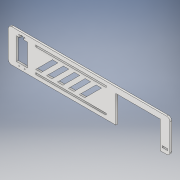
# Autodesk Inventor part: Cuerpo - LateralPrueba
Saved by Autodesk Inventor 2019 (Build 230136000, 136)
## iProperties
Created: 2020-02-14
Part Number: Cuerpo - LateralPrueba
Material: ABS Plastic
Document SubType Name: Modeling
Designer: Mafer1
Density: 1.06 g/cm^3
Appearance: Smooth - White
Mass: 36.6909 g
Surface Area: 287.559 cm^2
Volume: 34.614 cm^3
base_servo: 20.000 mm
altura_servo: 40.000 mm
agujero_servo: 2.000 mm
distancia_agujero_servo: 4.750 mm
largo_base: 200.000 mm
Author: Mafer1
Autodesk Inventor part; units mm, degrees
ref_plane "YZ Plane" through (0, 0, 0) normal (1, 0, 0) x (0, 1, 0)
ref_plane "XZ Plane" through (0, 0, 0) normal (0, 1, 0) x (-1, 0, 0)
ref_plane "XY Plane" through (0, 0, 0) normal (0, 0, 1) x (1, 0, 0)
sketch "Sketch7" plane through (0, 0, 0) normal (0, 0, 1) x (1, 0, 0)
  line L0 (296.3, 0) -> (296.3, 60.7)
  line L1 (296.3, 60.7) -> (0, 60.7)
  line L2 (0, 60.7) -> (0, 0)
  line L3 (50.3, 10) -> (179.25, 10)
  line L4 (179.25, 10) -> (179.25, 7)
  line L5 (179.25, 7) -> (50.3, 7)
  line L6 (50.3, 7) -> (50.3, 10)
  line L7 (15, 50.75) -> (35.3, 50.75)
  line L8 (35.3, 50.75) -> (35.3, 9.95)
  line L9 (35.3, 9.95) -> (15, 9.95)
  line L10 (15, 9.95) -> (15, 50.75)
  line L11 (50.3, 50.7) -> (179.25, 50.7)
  line L12 (179.25, 50.7) -> (179.25, 53.7)
  line L13 (179.25, 53.7) -> (50.3, 53.7)
  line L14 (50.3, 53.7) -> (50.3, 50.7)
  line L15 (0, 0) -> (197.25, 0)
  line L16 (197.25, 0) -> (197.25, 50.2)
  line L17 (197.25, 50.2) -> (278.3, 50.2)
  line L18 (278.3, 50.2) -> (278.3, 0)
  line L19 (278.3, 0) -> (296.3, 0)
  line L20 (282.3, 10) -> (292.3, 10)
  line L21 (292.3, 10) -> (292.3, 7)
  line L22 (292.3, 7) -> (282.3, 7)
  line L23 (282.3, 7) -> (282.3, 10)
  point P0 (50.3, 52.2)
  point P1 (50.3, 8.5)
  dimension "d154" = 128.95
  dimension "d159" = 3
  dimension "d161" = 40.8
  dimension "d162" = 20.3
  dimension "d163" = 15
  dimension "d168" = 7
  dimension "d224" = 40.7
  dimension "d225" = 15
  dimension "d232" = 60.7
  dimension "d233" = 7
  dimension "d234" = 18
  dimension "d235" = 81.05
  dimension "d236" = 9.95
  dimension "d237" = 10.5
  dimension "d239" = 18
  dimension "d240" = 4
  dimension "d247" = 10
  constraints: 48 end point, 9 parallel, 8 perpendicular, 5 horizontal, 2 equal length, 2 horizontal alignment, 2 midpoint, 1 point on line, 1 vertical alignment
  measures "d154" distance of L3.start L3.end
  measures "d159" distance between parallel lines of L5 L3
  measures "d161" distance of L7.end L8.end
  measures "d162" distance of L7.start L7.end
  measures "d163" distance between parallel lines of L10 L2
  measures "d168" distance between parallel lines of L13 L1
  measures "d224" distance between parallel lines of L3 L11
  measures "d225" distance from line of L8 point (50.3, 52.2)
  measures "d232" distance of L1.end L2.end
  measures "d233" distance between parallel lines of L15 L5
  measures "d234" distance between parallel lines of L16 L12
  measures "d235" distance of L16.end L17.end
  measures "d236" distance between parallel lines of L15 L9
  measures "d237" distance between parallel lines of L1 L17
  measures "d239" distance between parallel lines of L0 L18
  measures "d240" distance between parallel lines of L18 L23
  measures "d247" distance of L21.end L22.end
extrude "Extrusion7" add sketch "Sketch7" along normal blind 3.3 contours L19 L18 L17 L16 L15 L2 L1 L0 | L20 L21 L22 L23
fillet "Fillet1" radius 6 4 edges at (0, 60.7, 1.65) (0, 0, 1.65) (296.3, 60.7, 1.65) (296.3, 0, 1.65)
sketch "Sketch9" plane through (0, 0, 3.3) normal (0, 0, 1) x (1, 0, 0)
  arc A0 (290.3, 0) -> (296.3, 6) centre (290.3, 6) ccw projected
  line L0 (296.3, 6) -> (296.3, 54.7) projected
  arc A1 (296.3, 54.7) -> (290.3, 60.7) centre (290.3, 54.7) ccw projected
  line L1 (290.3, 60.7) -> (6, 60.7) projected
  arc A2 (6, 60.7) -> (0, 54.7) centre (6, 54.7) ccw projected
  line L2 (0, 54.7) -> (0, 6) projected
  arc A3 (0, 6) -> (6, 0) centre (6, 6) ccw projected
  line L3 (35.3, 50.75) -> (35.3, 9.95) projected
  line L4 (35.3, 9.95) -> (15, 9.95) projected
  line L5 (15, 9.95) -> (15, 50.75) projected
  line L6 (15, 50.75) -> (35.3, 50.75) projected
  line L7 (50.3, 50.7) -> (50.3, 53.7) projected
  line L8 (50.3, 53.7) -> (179.25, 53.7) projected
  line L9 (179.25, 53.7) -> (179.25, 50.7) projected
  line L10 (179.25, 50.7) -> (50.3, 50.7) projected
  line L11 (179.25, 10) -> (179.25, 7) projected
  line L12 (179.25, 7) -> (50.3, 7) projected
  line L13 (50.3, 7) -> (50.3, 10) projected
  line L14 (50.3, 10) -> (179.25, 10) projected
  line L15 (50.3, 15) -> (81, 45.7)
  line L16 (81, 45.7) -> (91, 45.7)
  line L17 (91, 45.7) -> (60.3, 15)
  line L18 (60.3, 15) -> (50.3, 15)
  line L19 (6, 0) -> (197.25, 0) projected
  line L20 (197.25, 0) -> (197.25, 50.2) projected
  line L21 (197.25, 50.2) -> (278.3, 50.2) projected
  line L22 (278.3, 50.2) -> (278.3, 0) projected
  line L23 (278.3, 0) -> (290.3, 0) projected
  point P0 (0, 0)
  dimension "d172" = 45
  dimension "d173" = 10
  dimension "d175" = 5
  dimension "d182" = 5
  constraints: 8 end point, 2 parallel, 1 horizontal, 1 vertical alignment
  measures "d172" angle of L18 L17
  measures "d173" distance of L15.end L16.end
  measures "d175" distance between parallel lines of L10 L16
  measures "d182" distance between parallel lines of L18 L14
extrude "Extrusion8" cut sketch "Sketch9" against normal blind 3.3 contours L15 L16 L17 L18
sketch "Sketch10" plane through (0, 0, 3.3) normal (0, 0, 1) x (1, 0, 0)
  line L0 (15, 9.95) -> (15, 50.75) projected
  line L1 (15, 50.75) -> (35.3, 50.75) projected
  line L2 (35.3, 50.75) -> (35.3, 9.95) projected
  line L3 (35.3, 9.95) -> (15, 9.95) projected
  circle A0 centre (20, 54.7) radius 0.85
  circle A1 centre (30, 54.7) radius 0.85
  circle A2 centre (20, 5.2) radius 0.85
  circle A3 centre (30, 5.2) radius 0.85
  point P0 (0, 0)
  dimension "d183" = 1.7
  dimension "d184" = 5
  dimension "d185" = 10
  dimension "d186" = 5
  dimension "d187" = 10
  dimension "d188" = 3.95
  dimension "d189" = 4.75
  constraints: 4 centre point, 3 equal radius, 2 horizontal alignment
  measures "d183" diameter of A0
  measures "d184" distance from line of L0 A0.centre
  measures "d185" distance of A1.centre A0.centre
  measures "d186" distance from line of L0 A2.centre
  measures "d187" distance of A3.centre A2.centre
  measures "d188" distance from line of L1 A0.centre
  measures "d189" distance from line of L3 A2.centre
extrude "Extrusion9" cut sketch "Sketch10" against normal blind 10 contours A0 | A1 | A2 | A3
sketch "Sketch11" plane through (0, 0, 3.3) normal (0, 0, 1) x (1, 0, 0)
  line L0 (15, 50.75) -> (35.3, 50.75) projected
  line L1 (21.4, 55.85) -> (28.6, 55.85) construction
  line L2 (28.6, 55.85) -> (28.6, 50.75) construction
  line L3 (28.6, 50.75) -> (21.4, 50.75)
  line L4 (21.4, 50.75) -> (21.4, 55.85) construction
  line L5 (15, 9.95) -> (15, 50.75) projected
  line L6 (35.3, 50.75) -> (35.3, 9.95) projected
  line L7 (259.7, 10) -> (259.7, 50.8) projected
  line L8 (21.4, 53.25) -> (23.2205, 55.85)
  line L9 (26.7795, 55.85) -> (28.6, 53.25)
  line L10 (21.4, 50.75) -> (21.4, 53.25)
  line L11 (23.2205, 55.85) -> (26.7795, 55.85)
  line L12 (28.6, 53.25) -> (28.6, 50.75)
  point P0 (0, 0)
  dimension "d203" = 6.4
  dimension "d205" = 5.1
  dimension "d206" = 7.2
  dimension "d215" = 35
  dimension "d216" = 2.5
  dimension "d217" = 35
  constraints: 18 end point, 5 point on line, 2 collinear, 2 horizontal, 2 parallel, 1 equal length, 1 perpendicular
  measures "d203" distance between parallel lines of L5 L4
  measures "d205" distance between parallel lines of L0 L1
  measures "d206" distance of L1.start L1.end
  measures "d215" angle of L4 L8
  measures "d216" distance from line of L0 L8.start
  measures "d217" angle of L2 L9
extrude "Extrusion10" cut sketch "Sketch11" against normal blind 10
sketch "Sketch13" plane through (0, 0, 3.3) normal (0, 0, 1) x (1, 0, 0)
  line L0 (282.3, 10) -> (292.3, 10) projected
  line L1 (292.3, 10) -> (292.3, 7) projected
  line L2 (292.3, 7) -> (282.3, 7) projected
  line L3 (282.3, 7) -> (282.3, 10) projected
  point P0 (0, 0)
extrude "Extrusion11" cut sketch "Sketch13" against normal up to surface (3.3 mm away)
pattern_linear "Rectangular Pattern2" count 5 spacing 20 along (1, 0, 0) of "Extrusion8"
equation "\"base_servo\" = 20"
equation "\"altura_servo\" = 40"
equation "\"agujero_servo\" = 2"
equation "\"distancia_agujero_servo\" = 4.75"
equation "\"largo_base\" = 200"
body "Solid2"
